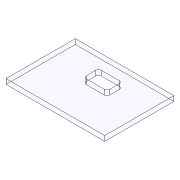
# Autodesk Inventor part: Lidar Sensor Case 4 v2
Saved by Autodesk Inventor 2018.3 (Build 223284000, 284)
## iProperties
Created: 2019-03-08
Part Number: Lidar Sensor Case 4 v2
Material: Generic
Document SubType Name: Modeling
Designer: aye06091
Mass: 6.90849 g
Surface Area: 53.3872 cm^2
Volume: 6.90849 cm^3
Density: 1 g/cm^3
Appearance: Clear - Blue
Author: aye06091
Autodesk Inventor part; units mm, degrees
ref_plane "YZ Plane" through (0, 0, 0) normal (1, 0, 0) x (0, 1, 0)
ref_plane "XZ Plane" through (0, 0, 0) normal (0, 1, 0) x (-1, 0, 0)
ref_plane "XY Plane" through (0, 0, 0) normal (0, 0, 1) x (1, 0, 0)
sketch "Sketch1" plane through (0, 0, 0) normal (0, 1, 0) x (-1, 0, 0)
  line L0 (0, 0) -> (-58.801, 0)
  line L1 (-58.801, 0) -> (-58.801, 41.275)
  line L2 (-58.801, 41.275) -> (0, 41.275)
  line L3 (0, 41.275) -> (0, 0)
  dimension "d0" = 41.275
  dimension "d1" = 58.801
  constraints: 8 end point, 2 parallel, 1 horizontal, 1 perpendicular
  measures "d0" distance of L2.end L0.start
  measures "d1" distance of L0.start L0.end
extrude "Extrusion1" add sketch "Sketch1" against normal blind 2.9972
sketch "Sketch2" plane through (0, 0, 0) normal (0, 1, 0) x (1, 0, 0)
  line L0 (0, -41.275) -> (0, 0) projected
  line L1 (58.801, -41.275) -> (0, -41.275) projected
  line L2 (22.4155, -8.5725) -> (36.3855, -8.5725)
  line L3 (36.3855, -8.5725) -> (36.3855, -17.4625)
  line L4 (36.3855, -17.4625) -> (22.4155, -17.4625)
  line L5 (22.4155, -17.4625) -> (22.4155, -8.5725)
  point P0 (29.4005, -13.0175)
  dimension "d7" = 8.89
  dimension "d17" = 13.97
  dimension "d22" = 6.985
  dimension "d23" = 4.445
  dimension "d24" = 29.4005
  dimension "d26" = 28.2575
  constraints: 8 end point, 2 parallel, 1 horizontal, 1 perpendicular
  measures "d7" distance of L2.end L3.end
  measures "d17" distance of L2.start L2.end
  measures "d22" distance from line of L5 point (29.401, -13.017)
  measures "d23" distance from line of L4 point (29.401, -13.017)
  measures "d24" distance from line of L0 point (29.401, -13.017)
  measures "d26" distance from line of L1 point (29.401, -13.017)
extrude "Extrusion2" cut sketch "Sketch2" against normal blind 2.9972
fillet "Fillet1" radius 1.5875 4 edges at (22.4155, -1.4986, 8.5725) (22.4155, -1.4986, 17.4625) (36.3855, -1.4986, 17.4625) (36.3855, -1.4986, 8.5725)
body "Solid1"
